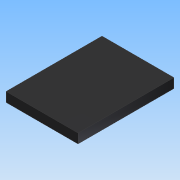
# Autodesk Inventor part: DRV8834
Saved by Autodesk Inventor 2015 (Build 190159000, 159)
## iProperties
Created: 2015-09-07
Part Number: DRV8834
Material: Generisch
Document SubType Name: Modeling
Designer: Johann
Density: 1 g/cm^3
Appearance: Gummi - schwarz
Mass: 0.619354 g
Surface Area: 7.61594 cm^2
Volume: 0.619354 cm^3
Author: Johann
Autodesk Inventor part; units mm, degrees
ref_plane "YZ Plane" through (0, 0, 0) normal (1, 0, 0) x (0, 1, 0)
ref_plane "XZ Plane" through (0, 0, 0) normal (0, 1, 0) x (-1, 0, 0)
ref_plane "XY Plane" through (0, 0, 0) normal (0, 0, 1) x (1, 0, 0)
sketch "Skizze1" plane through (0, 0, 0) normal (0, 0, 1) x (1, 0, 0)
  line L0 (-7.62, -10.16) -> (7.62, -10.16)
  line L1 (7.62, -10.16) -> (7.62, 10.16)
  line L2 (7.62, 10.16) -> (-7.62, 10.16)
  line L3 (-7.62, 10.16) -> (-7.62, -10.16)
  line L4 (-7.62, -10.16) -> (7.62, 10.16) construction
  line L5 (7.62, -10.16) -> (-7.62, 10.16) construction
  point P0 (0, 0)
  dimension "d0" = 15.24
  dimension "d1" = 20.32
  constraints: 12 end point, 2 midpoint, 2 parallel, 1 horizontal, 1 perpendicular
  measures "d0" distance of L1.end L2.end
  measures "d1" distance of L0.end L1.end
extrude "Extrusion1" add sketch "Skizze1" along normal blind 2
